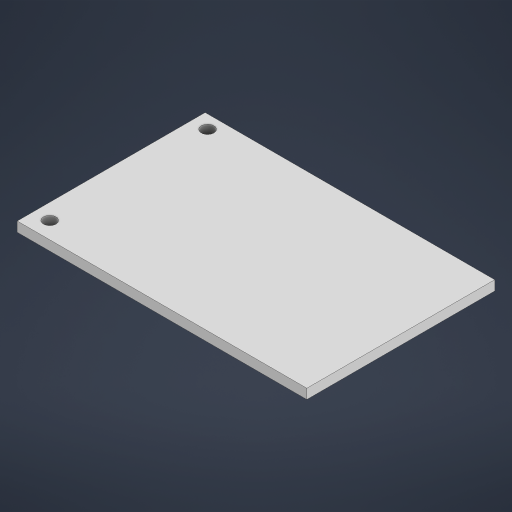
# Autodesk Inventor part: SD card holder
Saved by Autodesk Inventor 2023 (Build 270158000, 158)
## iProperties
Created: 2024-01-04
Part Number: SD card holder
Material: Generic
Document SubType Name: Modeling
Designer: nick_
Density: 1 g/cm^3
Appearance: Default
Author: nick_
Autodesk Inventor part; units mm, degrees
ref_plane "YZ Plane" through (0, 0, 0) normal (1, 0, 0) x (0, 1, 0)
ref_plane "XZ Plane" through (0, 0, 0) normal (0, 1, 0) x (-1, 0, 0)
ref_plane "XY Plane" through (0, 0, 0) normal (0, 0, 1) x (1, 0, 0)
sketch "Sketch1" plane through (0, 0, 0) normal (0, 1, 0) x (-1, 0, 0)
  line L0 (-23.765, 15.42) -> (23.765, 15.42)
  line L1 (23.765, 15.42) -> (23.765, -15.42)
  line L2 (23.765, -15.42) -> (-23.765, -15.42)
  line L3 (-23.765, -15.42) -> (-23.765, 15.42)
  line L4 (-23.765, 15.42) -> (23.765, -15.42) construction
  line L5 (23.765, 15.42) -> (-23.765, -15.42) construction
  point P0 (0, 0)
  dimension "d0" = 47.53
  dimension "d1" = 30.84
  constraints: 12 end point, 2 midpoint, 2 parallel, 1 horizontal, 1 perpendicular
  measures "d0" distance of L1.end L2.end
  measures "d1" distance of L0.end L1.end
extrude "Extrusion1" add sketch "Sketch1" along normal blind 1.6
sketch "Sketch2" plane through (0, 1.6, 0) normal (0, 1, 0) x (1, 0, 0)
  line L0 (23.765, 15.42) -> (-23.765, 15.42) projected
  line L1 (-23.765, -15.42) -> (23.765, -15.42) projected
  line L2 (-23.765, 15.42) -> (-23.765, -15.42) projected
  point P0 (0, 0)
  point P1 (-21.175, -12.68)
  point P2 (-21.175, 13.23)
  dimension "d4" = 25.91
  dimension "d5" = 2.19
  dimension "d6" = 2.74
  dimension "d7" = 2.59
  constraints: 1 vertical alignment
  measures "d4" distance of point (-21.175, 13.23) point (-21.175, -12.68)
  measures "d5" distance from line of L0 point (-21.175, 13.23)
  measures "d6" distance from line of L1 point (-21.175, -12.68)
  measures "d7" distance from line of L2 point (-21.175, 13.23)
hole "Hole1" at (-21.175, 1.6, 12.68) at (-21.175, 1.6, -13.23) direction (0, -1, 0) diameter 2.08 end through all
body "Solid1"
